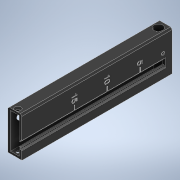
# Autodesk Inventor part: Magazin2
Saved by Autodesk Inventor 2021 (Build 250183000, 183)
## iProperties
Created: 2024-08-10
Part Number: Magazin2
Material: Generic
Document SubType Name: Modeling
Designer: Lukas
Density: 1 g/cm^3
Appearance: Default
Author: Lukas
Autodesk Inventor part; units mm, degrees
ref_plane "YZ Plane" through (0, 0, 0) normal (1, 0, 0) x (0, 1, 0)
ref_plane "XZ Plane" through (0, 0, 0) normal (0, 1, 0) x (-1, 0, 0)
ref_plane "XY Plane" through (0, 0, 0) normal (0, 0, 1) x (1, 0, 0)
sketch "Sketch1" plane through (0, 0, 0) normal (0, 0, 1) x (1, 0, 0)
  line L0 (-8, -22.5) -> (8, -22.5)
  line L1 (8, -22.5) -> (8, 20.7)
  line L2 (8, 20.7) -> (6.2, 22.5)
  line L3 (6.2, 22.5) -> (-6.2, 22.5)
  line L4 (-6.2, 22.5) -> (-8, 20.7)
  line L5 (-8, 20.7) -> (-8, -22.5)
  point P0 (0, 0)
  point P1 (0, 22.5)
  dimension "d0" = 45
  dimension "d1" = 16
  dimension "d2" = 1.8
  dimension "d3" = 22.5
  constraints: 12 end point, 3 perpendicular, 2 parallel, 1 horizontal, 1 horizontal alignment, 1 midpoint, 1 vertical alignment
  measures "d0" distance between parallel lines of L0 L3
  measures "d1" distance between parallel lines of L1 L5
  measures "d2" horizontal distance of L3.end L4.end
  measures "d3" distance from line of point (0, 0) L0
extrude "Extrusion1" add sketch "Sketch1" along normal blind 170
sketch "Sketch2" plane through (-8, -22.5, 0) normal (0, -1, 0) x (1, 0, 0)
  circle A0 centre (8, 7.75) radius 5
  line L0 (0, 0) -> (16, 0) projected
  point P0 (8, 0)
  point P1 (8, 0)
  dimension "d6" = 7.75
  dimension "d7" = 10
  constraints: 1 centre point, 1 midpoint, 1 vertical alignment
  measures "d6" distance from line of L0 A0.centre
  measures "d7" diameter of A0
extrude "Extrusion2" cut sketch "Sketch2" against normal through all
chamfer "Chamfer1" distance 1 distance2 2 1 edges at (-5, -22.5, 7.75) measured on face at (-5.5, -22.5, 7.75)
ref_plane "Work Plane1" through (-6.2, 2.4, 0) normal (0, 1, 0) x (1, 0, 0)
sketch "Sketch3" plane through (-6.2, 2.4, 0) normal (0, 1, 0) x (1, 0, 0)
  line L0 (-1.8, 0) -> (-1.8, -170) projected
  line L1 (-1.8, 0) -> (14.2, 0) projected
  arc A0 (-1.8, -11.75) -> (-1.8, -8.75) centre (-2.925, -10.25) ccw
  circle A1 centre (6.2, -7.75) radius 5 projected
  line L2 (-2.925, -10.25) -> (-2.925, -13.25)
  point P0 (6.2, 0)
  dimension "d14" = 0.75
  dimension "d15" = 3
  dimension "d16" = 2.5
  dimension "d17" = 3
  constraints: 2 end point, 2 point on circle, 2 point on line, 1 centre point, 1 vertical
  measures "d14" distance edge to line of A0 L0
  measures "d15" distance of A0.start A0.end
  measures "d16" vertical distance of L2.start A1.centre
  measures "d17" distance of L2.start L2.end
revolve "Revolution1" cut sketch "Sketch3" angle 360 about axis through (-9.125, 2.4, 10.25) along (0, 0, 1) contours A0 L0
fillet "Fillet1" radius 1 2 edges at (-8, 3.9, 10.25) (-8, 0.9, 10.25)
mirror "Mirror1" about plane through (0, 0, 0) normal (1, 0, 0) of "Revolution1", "Fillet1"
ref_plane "Work Plane2" through (0, 0, 7.75) normal (0, 0, -1) x (-1, 0, 0)
sketch "Sketch4" plane through (0, 0, 170) normal (0, 0, 1) x (1, 0, 0)
  line L0 (5, 20) -> (-5, 20)
  line L1 (-5, 20) -> (-5, -20)
  line L2 (-5, -20) -> (5, -20)
  line L3 (5, -20) -> (5, 20)
  point P0 (0, 0)
  point P1 (0, 20)
  point P2 (-5, 0)
  dimension "d20" = 40
  dimension "d21" = 10
  constraints: 8 end point, 2 midpoint, 2 parallel, 1 horizontal, 1 horizontal alignment, 1 perpendicular, 1 vertical alignment
  measures "d20" distance of L0.end L1.end
  measures "d21" distance of L0.start L0.end
extrude "Extrusion3" cut sketch "Sketch4" against normal up to surface (162.25 mm away)
sketch "Sketch5" plane through (-8, -22.5, 0) normal (0, -1, 0) x (1, 0, 0)
  circle A0 centre (8, 166.6) radius 1.6
  line L0 (0, 170) -> (16, 170) projected
  point P0 (8, 0)
  point P1 (8, 170)
  dimension "d25" = 3.2
  dimension "d26" = 3.4
  constraints: 1 centre point, 1 midpoint, 1 vertical alignment
  measures "d25" diameter of A0
  measures "d26" distance from line of L0 A0.centre
extrude "Extrusion4" cut sketch "Sketch5" against normal through all
sketch "Sketch6" plane through (-8, -22.5, 0) normal (1, 0, 0) x (0, 0, -1)
  line L0 (-140, 11.6) -> (-160, 31.6) construction
  line L1 (-137.8787, 13.7213) -> (-157.8787, 33.7213)
  line L2 (-162.1213, 29.4787) -> (-142.1213, 9.4787)
  arc A0 (-142.1213, 9.4787) -> (-137.8787, 13.7213) centre (-140, 11.6) ccw
  arc A1 (-157.8787, 33.7213) -> (-162.1213, 29.4787) centre (-160, 31.6) ccw
  line L3 (-170, 0) -> (-170, 43.2) projected
  point P0 (0, 22.5)
  point P1 (-150, 21.6)
  point P2 (-170, 21.6)
  dimension "d29" = 20
  dimension "d30" = 20
  dimension "d31" = 6
  dimension "d32" = 20
  constraints: 8 end point, 4 point on circle, 4 tangent, 2 centre point, 2 midpoint, 1 horizontal alignment, 1 parallel
  measures "d29" horizontal distance of L0.start L0.end
  measures "d30" horizontal distance of L0.start L0.end
  measures "d31" distance between parallel lines of L1 L2
  measures "d32" distance from line of L3 point (-150, 21.6)
extrude "Extrusion5" cut sketch "Sketch6" along normal up to surface (13 mm away)
pattern_linear "Rectangular Pattern1" count 7 spacing 20 along (0, 0, -1) of "Extrusion5"
sketch "Sketch7" plane through (0, 0, 170) normal (0, 0, 1) x (1, 0, 0)
  line L0 (8, -22.5) -> (8, 20.7) projected
  line L1 (8, -13) -> (6.5, -13)
  line L2 (6.5, -13) -> (6.5, -10.5)
  line L3 (6.5, -10.5) -> (5, -10.5)
  line L4 (5, 20) -> (5, -20) projected
  line L5 (5, -10.5) -> (5, -5.5)
  line L6 (5, -5.5) -> (6.5, -5.5)
  line L7 (6.5, -5.5) -> (6.5, -3)
  line L8 (6.5, -3) -> (8, -3)
  line L9 (8, -3) -> (8, -13)
  line L10 (5, -20) -> (-5, -20) projected
  point P0 (0, 0)
  point P1 (5, -8)
  dimension "d38" = 5
  dimension "d39" = 10
  dimension "d40" = 1.5
  dimension "d47" = 8
  constraints: 16 end point, 6 perpendicular, 4 point on line, 1 collinear, 1 midpoint, 1 vertical
  measures "d38" distance between parallel lines of L6 L3
  measures "d39" distance between parallel lines of L8 L1
  measures "d40" distance between parallel lines of L0 L2
  measures "d47" vertical distance of point (5, -8) point (0, 0)
extrude "Extrusion6" cut sketch "Sketch7" against normal up to surface (162.25 mm away)
chamfer "Chamfer2" distance 0.5 angle 45 4 edges at (6.5, -5.5, 88.875) (6.5, -10.5, 88.875) (6.5, -3, 88.875) (6.5, -13, 88.875)
sketch "Sketch8" plane through (8, -22.5, 0) normal (1, 0, 0) x (0, 0, -1)
  line L0 (-7.75, 19.5) -> (-170, 19.5) projected
  line L1 (-37, 19.5) -> (-36, 19.5)
  line L2 (-36, 19.5) -> (-36, 24.5)
  line L3 (-36, 24.5) -> (-37, 24.5)
  line L4 (-37, 24.5) -> (-37, 19.5)
  line L5 (-74, 19.5) -> (-73, 19.5)
  line L6 (-73, 19.5) -> (-73, 24.5)
  line L7 (-73, 24.5) -> (-74, 24.5)
  line L8 (-74, 24.5) -> (-74, 19.5)
  line L9 (-34, 34.5) -> (-34, 26.5) construction
  line L10 (-34, 26.5) -> (-39, 26.5) construction
  line L11 (-39, 26.5) -> (-39, 34.5) construction
  line L12 (-39, 34.5) -> (-34, 34.5) construction
  line L13 (-71, 34.5) -> (-71, 26.5) construction
  line L14 (-71, 26.5) -> (-76, 26.5) construction
  line L15 (-76, 26.5) -> (-76, 34.5) construction
  line L16 (-76, 34.5) -> (-71, 34.5) construction
  line L17 (-111, 19.5) -> (-110, 19.5)
  line L18 (-110, 19.5) -> (-110, 24.5)
  line L19 (-110, 24.5) -> (-111, 24.5)
  line L20 (-111, 24.5) -> (-111, 19.5)
  line L21 (-113, 34.5) -> (-108, 34.5) construction
  line L22 (-108, 34.5) -> (-108, 26.5) construction
  line L23 (-108, 26.5) -> (-113, 26.5) construction
  line L24 (-113, 26.5) -> (-113, 34.5) construction
  line L25 (-37.8377, 30.8125) -> (-37.7736, 30.0396)
  spline S0 degree 2 poles (-37.7736, 30.0396) (-38.3407, 29.9527) (-38.9078, 29.3308) (-38.9078, 28.8872) knots 0 0 0 1 2 2 2
  spline S1 degree 2 poles (-38.9078, 28.8872) (-38.9078, 28.3476) (-38.1029, 27.6159) (-37.4398, 27.6159) knots 0 0 0 1 2 2 2
  spline S2 degree 2 poles (-37.4398, 27.6159) (-36.8087, 27.6159) (-36.077, 28.3201) (-36.077, 28.8963) knots 0 0 0 1 2 2 2
  spline S3 degree 2 poles (-36.077, 28.8963) (-36.077, 29.253) (-36.4017, 29.8247) (-36.6623, 29.9893) knots 0 0 0 1 2 2 2
  line L26 (-36.6623, 29.9893) -> (-36.5709, 30.6799)
  line L27 (-36.5709, 30.6799) -> (-33.4886, 30.0991)
  line L28 (-33.4886, 30.0991) -> (-33.4886, 27.1174)
  line L29 (-33.4886, 27.1174) -> (-34.1928, 27.1174)
  line L30 (-34.1928, 27.1174) -> (-34.1928, 29.5091)
  line L31 (-34.1928, 29.5091) -> (-35.8026, 29.8338)
  spline S4 degree 2 poles (-35.8026, 29.8338) (-35.4276, 29.2942) (-35.4276, 28.6997) knots 0 0 0 1 1 1
  spline S5 degree 2 poles (-35.4276, 28.6997) (-35.4276, 27.9131) (-36.516, 26.8338) (-37.3712, 26.8338) knots 0 0 0 1 2 2 2
  spline S6 degree 2 poles (-37.3712, 26.8338) (-38.1898, 26.8338) (-38.7843, 27.3095) knots 0 0 0 1 1 1
  spline S7 degree 2 poles (-38.7843, 27.3095) (-39.5114, 27.8857) (-39.5114, 28.8826) knots 0 0 0 1 1 1
  spline S8 degree 2 poles (-39.5114, 28.8826) (-39.5114, 29.7012) (-38.5968, 30.7393) (-37.8377, 30.8125) knots 0 0 0 1 2 2 2
  line L32 (-76.4611, 32.7012) -> (-76.4611, 33.4375)
  line L33 (-76.4611, 33.4375) -> (-71.7691, 33.4375)
  spline S9 degree 2 poles (-71.7691, 33.4375) (-72.0206, 33.7027) (-72.5282, 34.5671) (-72.6563, 34.9101) knots 0 0 0 1 2 2 2
  line L34 (-72.6563, 34.9101) -> (-71.9428, 34.9101)
  spline S10 degree 2 poles (-71.9428, 34.9101) (-71.6547, 34.2927) (-70.827, 33.3689) (-70.4383, 33.1768) knots 0 0 0 1 2 2 2
  line L35 (-70.4383, 33.1768) -> (-70.4383, 32.7012)
  line L36 (-70.4383, 32.7012) -> (-76.4611, 32.7012)
  spline S11 degree 2 poles (-73.5023, 30.8125) (-72.4367, 30.8125) (-71.138, 30.3735) (-70.4383, 29.5137) (-70.4383, 28.8552) knots 0 0 0 1 2 3 3 3
  spline S12 degree 2 poles (-70.4383, 28.8552) (-70.4383, 28.375) (-70.827, 27.6433) (-71.5587, 27.1723) (-72.6105, 26.9024) (-73.5023, 26.9024) knots 0 0 0 1 2 3 4 4 4
  spline S13 degree 2 poles (-73.5023, 26.9024) (-74.5587, 26.9024) (-75.8575, 27.3369) (-76.5617, 28.2012) (-76.5617, 28.8552) knots 0 0 0 1 2 3 3 3
  spline S14 degree 2 poles (-76.5617, 28.8552) (-76.5617, 29.7241) (-75.9444, 30.218) knots 0 0 0 1 1 1
  spline S15 degree 2 poles (-75.9444, 30.218) (-75.1898, 30.8125) (-73.5023, 30.8125) knots 0 0 0 1 1 1
  spline S16 degree 2 poles (-73.5023, 30.0534) (-74.984, 30.0534) (-75.9581, 29.3628) (-75.9581, 28.8552) knots 0 0 0 1 2 2 2
  spline S17 degree 2 poles (-75.9581, 28.8552) (-75.9581, 28.3521) (-74.9794, 27.6616) (-73.5023, 27.6616) knots 0 0 0 1 2 2 2
  spline S18 degree 2 poles (-73.5023, 27.6616) (-72.0206, 27.6616) (-71.0465, 28.3521) (-71.0465, 28.8643) knots 0 0 0 1 2 2 2
  spline S19 degree 2 poles (-71.0465, 28.8643) (-71.0465, 29.372) (-71.4764, 29.6738) knots 0 0 0 1 1 1
  spline S20 degree 2 poles (-71.4764, 29.6738) (-72.0252, 30.0534) (-73.5023, 30.0534) knots 0 0 0 1 1 1
  line L37 (-113.4611, 32.7012) -> (-113.4611, 33.4375)
  line L38 (-113.4611, 33.4375) -> (-108.7691, 33.4375)
  spline S21 degree 2 poles (-108.7691, 33.4375) (-109.0206, 33.7027) (-109.5282, 34.5671) (-109.6563, 34.9101) knots 0 0 0 1 2 2 2
  line L39 (-109.6563, 34.9101) -> (-108.9428, 34.9101)
  spline S22 degree 2 poles (-108.9428, 34.9101) (-108.6547, 34.2927) (-107.827, 33.3689) (-107.4383, 33.1768) knots 0 0 0 1 2 2 2
  line L40 (-107.4383, 33.1768) -> (-107.4383, 32.7012)
  line L41 (-107.4383, 32.7012) -> (-113.4611, 32.7012)
  line L42 (-111.888, 30.8125) -> (-111.8239, 30.0396)
  spline S23 degree 2 poles (-111.8239, 30.0396) (-112.391, 29.9527) (-112.9581, 29.3308) (-112.9581, 28.8872) knots 0 0 0 1 2 2 2
  spline S24 degree 2 poles (-112.9581, 28.8872) (-112.9581, 28.3476) (-112.1532, 27.6159) (-111.4901, 27.6159) knots 0 0 0 1 2 2 2
  spline S25 degree 2 poles (-111.4901, 27.6159) (-110.859, 27.6159) (-110.1273, 28.3201) (-110.1273, 28.8963) knots 0 0 0 1 2 2 2
  spline S26 degree 2 poles (-110.1273, 28.8963) (-110.1273, 29.253) (-110.452, 29.8247) (-110.7127, 29.9893) knots 0 0 0 1 2 2 2
  line L43 (-110.7127, 29.9893) -> (-110.6212, 30.6799)
  line L44 (-110.6212, 30.6799) -> (-107.5389, 30.0991)
  line L45 (-107.5389, 30.0991) -> (-107.5389, 27.1174)
  line L46 (-107.5389, 27.1174) -> (-108.2431, 27.1174)
  line L47 (-108.2431, 27.1174) -> (-108.2431, 29.5091)
  line L48 (-108.2431, 29.5091) -> (-109.8529, 29.8338)
  spline S27 degree 2 poles (-109.8529, 29.8338) (-109.4779, 29.2942) (-109.4779, 28.6997) knots 0 0 0 1 1 1
  spline S28 degree 2 poles (-109.4779, 28.6997) (-109.4779, 27.9131) (-110.5663, 26.8338) (-111.4215, 26.8338) knots 0 0 0 1 2 2 2
  spline S29 degree 2 poles (-111.4215, 26.8338) (-112.2401, 26.8338) (-112.8346, 27.3095) knots 0 0 0 1 1 1
  spline S30 degree 2 poles (-112.8346, 27.3095) (-113.5617, 27.8857) (-113.5617, 28.8826) knots 0 0 0 1 1 1
  spline S31 degree 2 poles (-113.5617, 28.8826) (-113.5617, 29.7012) (-112.6471, 30.7393) (-111.888, 30.8125) knots 0 0 0 1 2 2 2
  point P0 (0, 22.5)
  point P1 (-36.5, 24.5)
  point P2 (-73.5, 24.5)
  point P3 (-36.5, 26.5)
  point P4 (-73.5, 26.5)
  point P5 (-110.5, 26.5)
  point P6 (-110.5, 24.5)
  dimension "d48" = 36.5
  dimension "d49" = 1
  dimension "d50" = 5
  dimension "d51" = 8
  dimension "d52" = 5
  dimension "d53" = 2
  dimension "d54" = 8
  dimension "d55" = 5
  dimension "d56" = 2
  dimension "d57" = 73.5
  dimension "d58" = 8
  dimension "d59" = 5
  dimension "d61" = 2
  dimension "d62" = 110.5
  dimension "d63" = 37
  dimension "d64" = 37
  constraints: 24 end point, 6 horizontal, 6 midpoint, 6 parallel, 4 equal length, 3 perpendicular, 3 point on line, 3 vertical alignment, 6 other
  measures "d48" horizontal distance of point (0, 22.5) point (-36.5, 24.5)
  measures "d49" distance of L2.end L3.end
  measures "d50" distance of L3.end L1.start
  measures "d51" distance of L9.start L9.end
  measures "d52" distance of L9.end L10.end
  measures "d53" distance from line of point (-36.5, 24.5) L10
  measures "d54" distance of L16.end L13.end
  measures "d55" distance of L13.end L14.end
  measures "d56" distance from line of point (-73.5, 24.5) L14
  measures "d57" horizontal distance of point (0, 22.5) point (-73.5, 24.5)
  measures "d58" distance of L21.end L22.end
  measures "d59" distance of L22.end L23.end
  measures "d61" distance from line of point (-110.5, 24.5) L23
  measures "d62" horizontal distance of point (0, 22.5) point (-110.5, 24.5)
  measures "d63" distance of point (-73.5, 24.5) point (-36.5, 24.5)
  measures "d64" distance of point (-110.5, 24.5) point (-73.5, 24.5)
extrude "Extrusion7" cut sketch "Sketch8" against normal blind 0.2
chamfer "Chamfer3" distance 1.8 angle 45 2 edges at (-1.6, 22.5, 166.6) (-1.6, -22.5, 166.6)
equation "\"d3\" = 0.5 * d0"
equation "\"d54\" = d51"
equation "\"d56\" = d53"
equation "\"d58\" = d60"
equation "\"d61\" = d56"
equation "\"d60\" = 8"
body "Solid1"
